Fan inlet hole cover_v2 (Autodesk Fusion 360 design; units mm, degrees)
Autodesk Fusion 360 part; units mm, degrees
sketch "Sketch1" plane through (0, 0, 0) normal (1, 0, 0) x (0, 1, 0)
  circle A0 centre (-25, 25) radius 2.975
  circle A1 centre (-25, 25) radius 5
  dimension "d1" = 5.95
  dimension "d4" = 10
  constraint concentric A0 A1
  measures "d1" diameter of A0
  measures "d4" diameter of A1
extrude "Extrude1" add sketch "Sketch1" along normal blind 5 contours A0
extrude "Extrude2" add sketch "Sketch1" against normal blind 2 contours A0 | A1
chamfer "Chamfer1" distance 2 angle 45 1 edges at (-2, -29.6616, 26.8081) measured on face at (-2, -27.3344, 24.5087)
